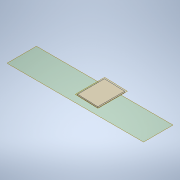
# Autodesk Inventor part: arc n°4
Saved by Autodesk Inventor 2020.2 (Build 242310000, 310)
## iProperties
Created: 2020-01-28
Part Number: arc n°4
Material: Générique
Document SubType Name: Modeling
Designer: anton
Density: 1 g/cm^3
Appearance: Par défaut
Author: anton
Autodesk Inventor part; units mm, degrees
ref_plane "YZ Plane" through (0, 0, 0) normal (1, 0, 0) x (0, 1, 0)
ref_plane "XZ Plane" through (0, 0, 0) normal (0, 1, 0) x (-1, 0, 0)
ref_plane "XY Plane" through (0, 0, 0) normal (0, 0, 1) x (1, 0, 0)
sketch "Esquisse1" plane through (0, 0, 0) normal (0, 0, 1) x (1, 0, 0)
  line L0 (-150.5839, 785.7) -> (150.5839, 785.7)
  arc A0 (150.5839, 785.7) -> (-150.5839, 785.7) centre (0, 0) ccw
  line L1 (-150.5839, 782.7) -> (150.5839, 782.7)
  arc A1 (150.5839, 782.7) -> (-150.5839, 782.7) centre (0, -3) ccw
  line L2 (-150.5839, 785.7) -> (-150.5839, 782.7)
  line L3 (150.5839, 785.7) -> (150.5839, 782.7)
  point P0 (0, 0)
  dimension "d4" = 785.7
  dimension "d8" = 3
  constraints: 8 end point, 4 point on circle, 2 centre point, 2 horizontal, 1 perpendicular
  measures "d4" distance from line of point (0, 0) L0
  measures "d8" distance between parallel lines of L0 L1
extrude "Extrusion1" add sketch "Esquisse1" along normal blind 65 contours A0 L0 A1 | L0 A1 L2 | L3 A1 L0
ref_plane "Plan de construction1" through (-150.5839, 782.7, 65) normal (0, -1, 0) x (0, 0, -1)
sketch "Esquisse2" plane through (-150.5839, 782.7, 65) normal (0, -1, 0) x (0, 0, -1)
  line L0 (0, 301.1678) -> (0, 0) projected
  line L1 (65, 301.1678) -> (65, 0) projected
  line L2 (0, 0) -> (65, 0)
  line L3 (65, 0) -> (65, 153)
  line L4 (65, 153) -> (0, 153)
  line L5 (0, 153) -> (0, 0)
  line L6 (0, 153) -> (65, 153)
  line L7 (65, 153) -> (65, 202)
  line L8 (65, 202) -> (0, 202)
  line L9 (0, 202) -> (0, 153)
  line L10 (0, 202) -> (65, 202)
  line L11 (65, 202) -> (65, 301.1678)
  line L12 (65, 301.1678) -> (0, 301.1678)
  line L13 (0, 301.1678) -> (0, 202)
  point P0 (65, 150.5839)
  point P1 (0, 153)
  point P2 (0, 202)
  dimension "d13" = 153
  dimension "d14" = 49
  constraints: 24 end point, 6 parallel, 3 horizontal, 3 perpendicular, 2 point on line
  measures "d13" distance between parallel lines of L2 L4
  measures "d14" distance between parallel lines of L8 L4
extrude "Extrusion2" cut sketch "Esquisse2" against normal through all contours L12 L1 L8 L0 | L4 L1 L2 L0
ref_plane "Plan de construction2" through (2.4161, 799.9964, 65) normal (0.0336609, 0.9994333, 0) x (0.9994333, -0.0336609, 0)
sketch "Esquisse3" plane through (2.4161, 799.9964, 65) normal (0.0336609, 0.9994333, 0) x (0.9994333, -0.0336609, 0)
  line L0 (0.101, 0) -> (0.101, 65) projected
  line L1 (49.1288, 65) -> (49.1288, 0) projected
  line L2 (0.101, 65) -> (49.1288, 65)
  line L3 (49.1288, 65) -> (49.1288, 0)
  line L4 (49.1288, 0) -> (0.101, 0)
  line L5 (0.101, 0) -> (0.101, 65)
  point P0 (24.5139, 65)
  point P1 (0.101, 0)
  point P2 (49.1288, 65)
  constraints: 8 end point, 2 parallel, 1 horizontal, 1 perpendicular
extrude "Extrusion3" cut sketch "Esquisse3" along normal blind 10
